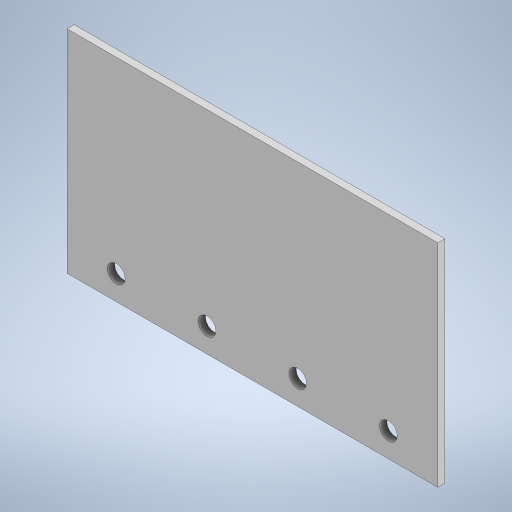
# Autodesk Inventor part: Front wall
Saved by Autodesk Inventor 2024.3 (Build 283343010, 343A)
## iProperties
Created: 2025-04-09
Part Number: Front wall
Material: Generic
Document SubType Name: Modeling
Designer: Vincent Larson
Density: 1 g/cm^3
Appearance: Default
Author: Vincent Larson
Autodesk Inventor part; units mm, degrees
ref_plane "YZ Plane" through (0, 0, 0) normal (1, 0, 0) x (0, 1, 0)
ref_plane "XZ Plane" through (0, 0, 0) normal (0, 1, 0) x (-1, 0, 0)
ref_plane "XY Plane" through (0, 0, 0) normal (0, 0, 1) x (1, 0, 0)
sketch "Sketch1" plane through (0, 0, 0) normal (0, 0, 1) x (1, 0, 0)
  line L0 (0, 0) -> (266.7, 0)
  line L1 (266.7, 0) -> (266.7, -152.4)
  line L2 (266.7, -152.4) -> (0, -152.4)
  line L3 (0, -152.4) -> (0, 0)
  dimension "d0" = 266.7
  dimension "d1" = 152.4
  constraints: 8 end point, 2 parallel, 1 horizontal, 1 perpendicular
  measures "d0" distance of L1.end L2.end
  measures "d1" distance of L0.end L1.end
extrude "Extrusion1" add sketch "Sketch1" along normal blind 5.08
sketch "Sketch2" plane through (0, 0, 5.08) normal (0, 0, 1) x (1, 0, 0)
  line L0 (0, -152.4) -> (266.7, -152.4) projected
  line L1 (59.8504, -152.4) -> (42.3244, -152.4)
  line L2 (0, 0) -> (0, -152.4) projected
  line L3 (266.7, -152.4) -> (266.7, 0) projected
  circle A0 centre (165.989, -134.874) radius 6.35
  circle A1 centre (231.267, -134.874) radius 6.35
  circle A2 centre (100.711, -134.874) radius 6.35
  circle A3 centre (35.433, -134.874) radius 6.35
  dimension "d9" = 12.7
  constraints: 4 centre point, 2 end point, 2 point on line
  measures "d9" diameter of A1
extrude "Extrusion2" cut sketch "Sketch2" against normal blind 8.382
body "Solid1"
